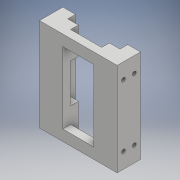
# Autodesk Inventor part: Spring support
Saved by Autodesk Inventor 2018 (Build 220112000, 112)
## iProperties
Created: 2019-06-06
Part Number: Spring support
Material: Generic
Document SubType Name: Modeling
Designer: aal_9
Density: 1 g/cm^3
Appearance: Default
Author: aal_9
Autodesk Inventor part; units mm, degrees
ref_plane "YZ Plane" through (0, 0, 0) normal (1, 0, 0) x (0, 1, 0)
ref_plane "XZ Plane" through (0, 0, 0) normal (0, 1, 0) x (-1, 0, 0)
ref_plane "XY Plane" through (0, 0, 0) normal (0, 0, 1) x (1, 0, 0)
sketch "Sketch1" plane through (0, 0, 0) normal (0, 1, 0) x (-1, 0, 0)
  line L0 (25, -30) -> (-25, -30)
  line L1 (-25, -30) -> (-25, 30)
  line L2 (-25, 30) -> (25, 30)
  line L3 (25, 30) -> (25, -30)
  point P0 (0, 0)
  dimension "d0" = 50
  dimension "d1" = 60
  dimension "d8" = 30
  dimension "d9" = 25
  constraints: 8 end point, 2 parallel, 1 horizontal, 1 perpendicular
  measures "d0" distance of L1.end L2.end
  measures "d1" distance of L2.end L0.start
  measures "d8" distance from line of point (0, 0) L2
  measures "d9" distance from line of point (0, 0) L3
extrude "Extrusion1" add sketch "Sketch1" along normal blind 15
sketch "Sketch2" plane through (0, 15, 0) normal (0, 1, 0) x (1, 0, 0)
  line L0 (-16.85, 12.5) -> (16.85, 12.5)
  line L1 (16.85, 12.5) -> (16.85, -12.5)
  line L2 (16.85, -12.5) -> (-16.85, -12.5)
  line L3 (-16.85, -12.5) -> (-16.85, 12.5)
  point P0 (0, 0)
  dimension "d4" = 33.7
  dimension "d5" = 25
  dimension "d6" = 12.5
  dimension "d7" = 16.85
  constraints: 8 end point, 2 parallel, 1 horizontal, 1 perpendicular
  measures "d4" distance of L1.end L2.end
  measures "d5" distance of L2.end L0.start
  measures "d6" distance from line of point (0, 0) L2
  measures "d7" distance from line of point (0, 0) L1
extrude "Extrusion2" cut sketch "Sketch2" against normal blind 10
sketch "Sketch3" plane through (0, 15, 0) normal (0, 1, 0) x (1, 0, 0)
  line L0 (-25, 30) -> (25, 30) projected
  line L1 (-25, -30) -> (25, -30) projected
  line L2 (-10, 30) -> (10, 30)
  line L3 (10, 30) -> (10, -30)
  line L4 (10, -30) -> (-10, -30)
  line L5 (-10, -30) -> (-10, 30)
  point P0 (0, 0)
  dimension "d12" = 20
  dimension "d13" = 10
  constraints: 8 end point, 2 parallel, 2 point on line, 1 horizontal, 1 perpendicular
  measures "d12" distance between parallel lines of L3 L5
  measures "d13" distance from line of point (0, 0) L3
extrude "Extrusion3" cut sketch "Sketch3" against normal up to surface (10 mm away)
sketch "Sketch4" plane through (0, 5, 0) normal (0, 1, 0) x (1, 0, 0)
  line L0 (-16.85, 12.5) -> (-10, 12.5) projected
  line L1 (16.85, -12.5) -> (10, -12.5) projected
  line L2 (10, 12.5) -> (10, 30) projected
  line L3 (-10, -30) -> (-10, -12.5) projected
  line L4 (10, 23) -> (-10, 23)
  line L5 (-10, 23) -> (-10, -23)
  line L6 (-10, -23) -> (10, -23)
  line L7 (10, -23) -> (10, 23)
  line L8 (-10, 30) -> (10, 30) projected
  line L9 (10, -30) -> (-10, -30) projected
  dimension "d18" = 7
  dimension "d19" = 7
  constraints: 8 end point, 2 parallel, 2 point on line, 1 horizontal, 1 perpendicular
  measures "d18" distance between parallel lines of L4 L8
  measures "d19" distance between parallel lines of L9 L6
extrude "Extrusion4" cut sketch "Sketch4" against normal up to next
sketch "Sketch6" plane through (-25, 0, -30) normal (-1, 0, 0) x (0, 0, 1)
  line L0 (0, 0) -> (0, 15) projected
  line L1 (60, 0) -> (60, 15) projected
  line L2 (60, 0) -> (0, 0) projected
  point P0 (30, 0)
  point P1 (10, 4)
  point P2 (50, 4)
  point P3 (50, 11)
  point P4 (10, 11)
  dimension "d24" = 7
  dimension "d25" = 7
  dimension "d26" = 10
  dimension "d27" = 10
  dimension "d28" = 10
  dimension "d29" = 10
  dimension "d30" = 4
  dimension "d31" = 4
  measures "d24" distance of point (10, 4) point (10, 11)
  measures "d25" distance of point (50, 4) point (50, 11)
  measures "d26" distance from line of L0 point (10, 11)
  measures "d27" distance from line of L1 point (50, 11)
  measures "d28" distance from line of L1 point (50, 4)
  measures "d29" distance from line of point (10, 4) L0
  measures "d30" distance from line of L2 point (10, 4)
  measures "d31" distance from line of L2 point (50, 4)
hole "Hole1" at (-25, 4, -20) at (-25, 4, 20) at (-25, 11, 20) at (-25, 11, -20) direction (1, 0, 0) diameter 2.459 depth 7 tip angle 118 thread size "M3x0.5" class "6H" standard "ANSI Metric M Profile"
sketch "Sketch7" plane through (25, 0, 30) normal (1, 0, 0) x (0, 0, -1)
  circle A0 centre (10, 4) radius 1.2295 projected
  circle A1 centre (10, 11) radius 1.2295 projected
  circle A2 centre (50, 11) radius 1.2295 projected
  circle A3 centre (50, 4) radius 1.2295 projected
  point P0 (30, 0)
  constraints: 4 coincident
hole "Hole2" at (25, 4, 20) at (25, 11, 20) at (25, 11, -20) at (25, 4, -20) direction (-1, 0, 0) diameter 2.459 depth 7 tip angle 118 thread size "M3x0.5" class "6H" standard "ANSI Metric M Profile"
sketch "Sketch8" plane through (-25, 0, 30) normal (0, 0, 1) x (1, 0, 0)
  line L0 (0, 15) -> (15, 15) projected
  line L1 (8.15, 15) -> (41.85, 15)
  line L2 (41.85, 15) -> (41.85, 10)
  line L3 (41.85, 10) -> (8.15, 10)
  line L4 (8.15, 10) -> (8.15, 15)
  line L5 (41.85, 15) -> (41.85, 5) projected
  line L6 (8.15, 15) -> (8.15, 5) projected
  point P0 (25, 0)
  dimension "d49" = 5
  dimension "d50" = 0
  dimension "d51" = 0
  dimension "d52" = 0
  constraints: 8 end point, 2 parallel, 1 horizontal, 1 perpendicular
  measures "d49" distance of L3.end L1.start
  measures "d50" distance between parallel lines of L0 L1
  measures "d51" distance between parallel lines of L5 L2
  measures "d52" distance between parallel lines of L6 L4
extrude "Extrusion6" cut sketch "Sketch8" against normal through all
body "Solid1"
